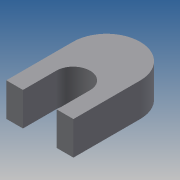
# Autodesk Inventor part: nub
Saved by Autodesk Inventor 2014 (Build 180170000, 170)
## iProperties
Created: 2014-01-24
Part Number: nub
Material: Generic
Document SubType Name: Modeling
Designer: Peele
Density: 1 g/cm^3
Appearance: Default
Author: Peele
Autodesk Inventor part; units mm, degrees
ref_plane "YZ Plane" through (0, 0, 0) normal (1, 0, 0) x (0, 1, 0)
ref_plane "XZ Plane" through (0, 0, 0) normal (0, 1, 0) x (-1, 0, 0)
ref_plane "XY Plane" through (0, 0, 0) normal (0, 0, 1) x (1, 0, 0)
sketch "Sketch1" plane through (0, 0, 0) normal (0, 0, 1) x (1, 0, 0)
  line L0 (-4.025, 0) -> (-4.025, -8)
  line L1 (-4.025, -8) -> (-2.025, -8)
  line L2 (-2.025, -8) -> (-2.025, -4)
  line L3 (2.025, -4) -> (2.025, -8)
  line L4 (2.025, -8) -> (4.025, -8)
  line L5 (4.025, -8) -> (4.025, 0)
  arc A0 (4.025, 0) -> (-4.025, 0) centre (0, 0) ccw
  arc A1 (2.025, -4) -> (-2.025, -4) centre (0, -4) ccw
  dimension "d0" = 4.05
  dimension "d1" = 8
  dimension "d3" = 2
  dimension "d4" = 4
  constraints: 12 end point, 4 point on circle, 4 tangent, 2 centre point, 2 equal length, 2 parallel, 2 perpendicular, 2 vertical, 1 coincident
  measures "d0" distance between parallel lines of L2 L3
  measures "d1" distance of L4.end L5.end
  measures "d3" distance of L3.end L4.end
  measures "d4" distance of L3.start L3.end
extrude "Extrusion1" add sketch "Sketch1" along normal blind 4
body "Solid1"
